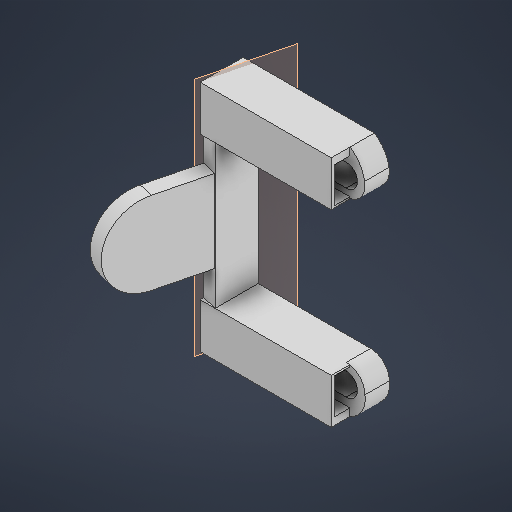
# Autodesk Inventor part: CapTurnerV3
Saved by Autodesk Inventor 2026 (Build 300175050, 175E)
## iProperties
Created: 2026-05-08
Part Number: CapTurnerV3
Material: Generic
Document SubType Name: Modeling
Designer: sniel
Density: 1 g/cm^3
Appearance: Default
Author: sniel
Autodesk Inventor part; units mm, degrees
ref_plane "YZ Plane" through (0, 0, 0) normal (1, 0, 0) x (0, 1, 0)
ref_plane "XZ Plane" through (0, 0, 0) normal (0, 1, 0) x (-1, 0, 0)
ref_plane "XY Plane" through (0, 0, 0) normal (0, 0, 1) x (1, 0, 0)
sketch "Sketch1" plane through (0, 0, 0) normal (0, 0, 1) x (1, 0, 0)
  circle A0 centre (-35, 5) radius 2.5
  circle A1 centre (-35, -43.3013) radius 2.5
  circle A2 centre (-5, -43.3013) radius 2.5
  circle A3 centre (-5, 5) radius 2.5
  circle A4 centre (-5, 5) radius 3
  circle A5 centre (-35, 5) radius 3
  circle A6 centre (-5, -43.3013) radius 3
  circle A7 centre (-5, 5) radius 5
  line L0 (-5, 8) -> (-35, 8)
  line L1 (-5, 2) -> (-35, 2)
  circle A8 centre (-35, -43.3013) radius 5
  circle A9 centre (-5, -43.3013) radius 5
  circle A10 centre (-35, -43.3013) radius 3
  line L2 (-5, -40.3013) -> (-35, -40.3013)
  line L3 (-5, -46.3013) -> (-35, -46.3013)
  circle A11 centre (-35, 5) radius 5
  line L4 (-35, 8) -> (-39, 8)
  line L5 (-35, 2) -> (-39, 2)
  line L6 (-35, -40.3013) -> (-39, -40.3013)
  line L7 (-35, -46.3013) -> (-39, -46.3013)
  line L8 (-5, 10) -> (-35, 10)
  line L9 (-5, 0) -> (-35, 0)
  line L10 (-5, -38.3013) -> (-35, -38.3013)
  line L11 (-5, -48.3013) -> (-35, -48.3013)
  line L12 (-35, 0) -> (-35, -38.3013)
  line L13 (-39, 2) -> (-39, -40.3013)
  point P0 (0, 0)
  dimension "d0" = 6
  dimension "d1" = 6
  dimension "d3" = 6
  dimension "d4" = 10
  dimension "d5" = 10
  dimension "d6" = 6
  dimension "d7" = 10
  constraints: 28 end point, 22 point on circle, 12 centre point, 9 coincident, 8 tangent, 5 horizontal, 2 parallel, 2 vertical
  measures "d0" diameter of A4
  measures "d1" diameter of A5
  measures "d3" diameter of A6
  measures "d4" diameter of A8
  measures "d5" diameter of A9
  measures "d6" diameter of A10
  measures "d7" diameter of A11
extrude "Extrusion1" add sketch "Sketch1" along normal blind 6.5 contours A4 L0 A7 L1 | L0 A11 L8 A7 | A7 L9 A11 L1 | L0 L4 A11 | A11 L5 L1 | L12 A8 L13 A11 | A8 L2 L6 | L10 A9 L2 A8 | A9 L3 A6 L2 | L7 L3 A8 | A8 L3 A9 L11 picked at (-7.4012, 8.2796) picked at (-7.4012, -46.5809)
sketch "Sketch2" plane through (-35, -38.3013, 0) normal (1, 0, 0) x (0, 0, -1)
  line L0 (-6.5, 0) -> (-6.5, 38.3013) projected
  line L1 (-6.5, 38.3013) -> (-6.5, 40.3013)
  line L2 (-6.5, 38.3013) -> (-11.5, 38.3013)
  line L3 (-6.5, 38.3013) -> (-1.5, 38.3013) construction
  line L4 (-6.5, 0) -> (-11.5, 0)
  line L5 (-6.5, 40.3013) -> (-6.5, -2) projected
  line L6 (-6.5, 0) -> (-1.5, 0) construction
  line L7 (-11.5, 0) -> (-11.5, 38.3013)
  point P0 (0, 38.3013)
  dimension "d10" = 5
  dimension "d11" = 180
  dimension "d12" = 5
  dimension "d13" = 180
  constraints: 12 end point, 3 horizontal, 2 collinear, 1 perpendicular
  measures "d10" distance of L0.end L2.end
  measures "d11" angle of L2 L3
  measures "d12" distance of L0.start L4.end
  measures "d13" angle of L4 L6
extrude "Extrusion2" add sketch "Sketch2" against normal blind 4
sketch "Sketch3" plane through (-35, -38.3013, 6.5) normal (0, -1, 0) x (1, 0, 0)
  line L0 (0, 5) -> (0, 0) projected
  line L1 (0, 5) -> (-4, 5) projected
  line L2 (-4, 0) -> (-4, 5) projected
  line L3 (0, 0) -> (-4, 0) projected
  line L4 (-4, 5) -> (-4, 4)
  line L5 (-4, 4) -> (0, 5)
  point P0 (35, -6.5)
  dimension "d16" = 1
  constraints: 4 end point, 1 point on line
  measures "d16" distance of L1.end L4.end
extrude "Extrusion3" cut sketch "Sketch3" against normal up to surface (38.3013 mm away) contours L5 L2 L1
ref_plane "Work Plane1" through (-39, -18.1506, 10.5) normal (0.9701, 0, 0.2425) x (0, 1, 0)
sketch "Sketch5" plane through (-35, -38.3013, 0) normal (1, 0, 0) x (0, 0, -1)
  line L0 (0, 38.3013) -> (0, 48.3013) projected
  line L1 (0, 48.3013) -> (-6.5, 48.3013) projected
  line L2 (-6.5, 38.3013) -> (-6.5, 48.3013) projected
  line L3 (0, 38.3013) -> (-6.5, 38.3013) projected
  line L4 (0, -10) -> (0, 0) projected
  line L5 (0, 0) -> (-6.5, 0) projected
  line L6 (-6.5, -10) -> (-6.5, 0) projected
  line L7 (0, -10) -> (-6.5, -10) projected
  line L8 (0, 0) -> (0, 38.3013) projected
  line L9 (0, 38.3013) -> (-6.5, 38.3013) projected
  line L10 (-6.5, 38.3013) -> (-11.5, 38.3013) projected
  line L11 (-11.5, 38.3013) -> (-11.5, 0) projected
  line L12 (-11.5, 0) -> (-6.5, 0) projected
  line L13 (0, 0) -> (-6.5, 0) projected
  line L14 (0, 48.3013) -> (0, 50.3013)
  line L15 (0, 50.3013) -> (-17.5997, 50.3013)
  line L16 (0, -10) -> (0, -12)
  line L17 (0, -12) -> (-16.7586, -12)
  line L18 (-11.5, 0) -> (-11.5, -14.3259)
  line L19 (-6.5, 38.3013) -> (-11.5, 38.3013) projected
  line L20 (-11.5, 38.3013) -> (-11.5, 54.2478)
  line L21 (-6.5, 48.3013) -> (-17.5997, 48.3013)
  line L22 (-6.5, -8) -> (-6.5, -10) projected
  line L23 (-6.5, -10) -> (-16.7586, -10)
  line L24 (-6.5, 38.3013) -> (-6.5, 38.8013)
  line L25 (-6.5, 38.8013) -> (-12, 38.8013)
  line L26 (-6.5, 0) -> (-6.5, -2) projected
  line L27 (-6.5, 0) -> (-6.5, -0.5)
  line L28 (-6.5, -0.5) -> (-13.9811, -0.5)
  line L29 (-11.5, 38.3013) -> (-10.5, 38.3013)
  line L30 (-10.5, 38.3013) -> (-10.5, 53.5621)
  line L31 (-11.5, 38.3013) -> (-11.5, 0) projected
  line L32 (-11.5, 0) -> (-10.5, 0)
  line L33 (-10.5, 0) -> (-10.5, -14.7859)
  point P0 (0, 38.3013)
  point P1 (-10.5, -0.5)
  point P2 (-6.5, -0.5)
  point P3 (-11.5, -12)
  point P4 (-10.5, -10)
  point P5 (-11.5, 50.3013)
  point P6 (-10.5, 38.8013)
  point P7 (-10.5, 48.3013)
  dimension "d26" = 2
  dimension "d27" = 2
  dimension "d28" = 0.5
  dimension "d29" = 90
  dimension "d30" = 0.5
  dimension "d31" = 1
  constraints: 32 end point, 5 vertical, 4 perpendicular, 4 point on line, 2 horizontal
  measures "d26" distance of L0.end L14.end
  measures "d27" distance of L4.start L16.end
  measures "d28" distance of L9.end L24.end
  measures "d29" angle of L25 L24
  measures "d30" distance of L5.end L27.end
  measures "d31" distance of L10.end L29.end
extrude "Extrusion5" add sketch "Sketch5" along normal blind 31 and the other way blind 4 contours L1 L21 L30 L15 L14 | L10 L30 L25 L2 | L10 L20 L25 L30 | L16 L17 L33 L23 L7 | L6 L28 L33 L12 | L30 L25 L20 L21 | L21 L20 L15 L30 | L33 L28 L18 L12 | L33 L17 L18 L23 | L23 L18 L28 L33
sketch "Sketch24" plane through (0, 0, 0) normal (0, 0, -1) x (-1, 0, 0)
  line L0 (39, 2) -> (39, -40.3013) projected
  line L1 (5, 2) -> (39, 2) projected
  arc A0 (5, 8) -> (5, 2) centre (5, 5) ccw projected
  line L2 (39, 8) -> (5, 8) projected
  arc A1 (39, 8) -> (35, 10) centre (35, 5) ccw projected
  line L3 (39, 10) -> (35, 10) projected
  line L4 (39, 12) -> (39, 10) projected
  line L5 (4, 12) -> (39, 12) projected
  line L6 (4, 10) -> (4, 12) projected
  line L7 (5, 10) -> (4, 10) projected
  arc A2 (5, 10) -> (5, 0) centre (5, 5) ccw projected
  line L8 (35, 0) -> (5, 0) projected
  line L9 (35, -38.3013) -> (35, 0) projected
  line L10 (5, -38.3013) -> (35, -38.3013) projected
  arc A3 (5, -38.3013) -> (5, -48.3013) centre (5, -43.3013) ccw projected
  line L11 (5, -48.3013) -> (4, -48.3013) projected
  line L12 (4, -50.3013) -> (4, -48.3013) projected
  line L13 (39, -50.3013) -> (4, -50.3013) projected
  line L14 (39, -48.3013) -> (39, -50.3013) projected
  line L15 (39, -48.3013) -> (35, -48.3013) projected
  arc A4 (35, -48.3013) -> (39, -46.3013) centre (35, -43.3013) ccw projected
  line L16 (5, -46.3013) -> (39, -46.3013) projected
  arc A5 (5, -40.3013) -> (5, -46.3013) centre (5, -43.3013) ccw projected
  line L17 (39, -40.3013) -> (5, -40.3013) projected
  line L18 (4, 12) -> (4, 0) projected
  arc A6 (4, 12) -> (0, 5) centre (8.7961, 4.6165) ccw
  arc A7 (0, -43.3013) -> (4, -50.3013) centre (6.6386, -44.1506) ccw
  line L19 (39, 8) -> (39, 12)
  line L20 (39, 0.5) -> (4, 0.5) projected
  line L21 (39, -46.3013) -> (39, -48.3982)
  line L22 (39, -48.3013) -> (39, -50.3013) projected
  point P0 (0, 0)
  point P1 (0.101, 6)
  constraints: 6 point on circle, 4 end point, 2 centre point, 1 perpendicular, 1 point on line
extrude "Extrusion23" add sketch "Sketch24" against normal blind 6.5 contours L18 L7 A2 | A2 A6 L6 L18 | L21 L15 A4 | A1 L3 L19 | A3 L11 L12 A7
sketch "Sketch25" plane through (-39, 2, 0) normal (-1, 0, 0) x (0, 0, 1)
  line L0 (6.5, -50.3013) -> (10.5, -50.3013) projected
  line L1 (10.5, -50.3013) -> (10.5, -40.8013) projected
  line L2 (10.5, -40.8013) -> (6.5, -40.8013) projected
  line L3 (6.5, -40.8013) -> (6.5, -50.3013)
  line L4 (0, -45.3013) -> (10.5, -45.3013) projected
  line L5 (6.5, -42.3013) -> (0, -42.3013) projected
  line L6 (0, 0) -> (0, -42.3013) projected
  point P0 (0, -2)
  point P1 (6.5, -45.3013)
  constraints: 2 end point, 1 perpendicular
extrude "Extrusion24" cut sketch "Sketch25" against normal blind 23.75
sketch "Sketch35" plane through (-39, -18.1506, 10.5) normal (0.9701, 0, 0.2425) x (0, 1, 0)
  line L0 (-20.1506, 0) -> (18.1506, 0) projected
  line L1 (0, 0) -> (0, 30)
  line L2 (0, 0) -> (30, 0) construction
  circle A0 centre (0, 14) radius 11
  line L3 (11, 14) -> (11, 0)
  line L4 (-11, 14) -> (-11, 0)
  line L5 (0, 25) -> (0, 35)
  point P0 (18.1506, -19.6454)
  point P1 (11, 0)
  dimension "d177" = 30
  dimension "d178" = 90
  dimension "d179" = 22
  dimension "d182" = 10
  constraints: 10 end point, 6 point on line, 4 perpendicular, 3 point on circle, 1 centre point, 1 horizontal, 1 tangent
  measures "d177" distance of L1.start L1.end
  measures "d178" angle of L2 L1
  measures "d179" diameter of A0
  measures "d182" distance of L5.start L5.end
extrude "Extrusion34" add sketch "Sketch35" along normal blind 4
body "Solid1"
